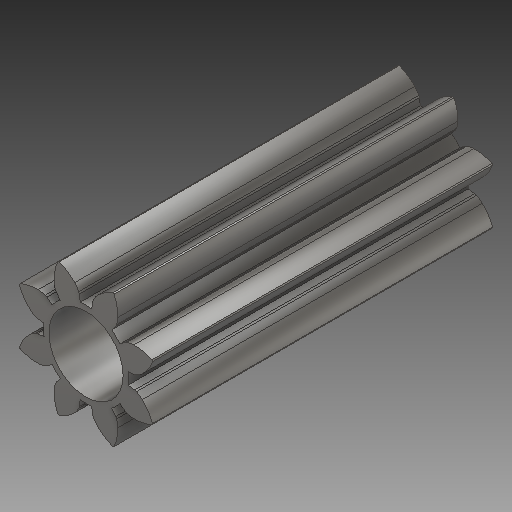
# Autodesk Inventor part: ピニオン8
Saved by Autodesk Inventor 2020 (Build 240168000, 168)
## iProperties
Created: 2018-09-09
Part Number: ピニオン8
Material: 鋼、炭素鋼
Document SubType Name: Modeling
Designer: 雪村
Density: 7.85 g/cm^3
Appearance: 半つや出し
Mass: 0.86128 g
Surface Area: 4.58108 cm^2
Volume: 0.109717 cm^3
Author: 雪村
Autodesk Inventor part; units mm, degrees
ref_plane "YZ Plane" through (0, 0, 0) normal (1, 0, 0) x (0, 1, 0)
ref_plane "XZ Plane" through (0, 0, 0) normal (0, 1, 0) x (-1, 0, 0)
ref_plane "XY Plane" through (0, 0, 0) normal (0, 0, 1) x (1, 0, 0)
sketch "スケッチ1" plane through (0, 0, 0) normal (0, 0, 1) x (1, 0, 0)
  arc A0 (-4.3849, 83.0601) -> (-4.408, 82.9909) centre (-4.1206, 82.9335) ccw
  arc A1 (-4.2334, 83.2827) -> (-4.3849, 83.0601) centre (-3.6288, 82.7082) ccw
  arc A2 (-3.6386, 83.6726) -> (-4.2334, 83.2827) centre (-3.1026, 82.2065) ccw
  arc A3 (-5.8318, 82.6909) -> (-5.7992, 82.6257) centre (-5.5555, 82.7883) ccw
  arc A4 (-5.8821, 82.9554) -> (-5.8318, 82.6909) centre (-5.0484, 82.9767) ccw
  arc A5 (-5.7372, 83.6517) -> (-5.8821, 82.9554) centre (-4.3215, 82.994) ccw
  arc A6 (-6.5939, 81.4067) -> (-6.5247, 81.3836) centre (-6.4673, 81.6709) ccw
  arc A7 (-6.8165, 81.5582) -> (-6.5939, 81.4067) centre (-6.242, 82.1627) ccw
  arc A8 (-7.2064, 82.153) -> (-6.8165, 81.5582) centre (-5.7403, 82.6889) ccw
  arc A9 (-6.2247, 79.9597) -> (-6.1595, 79.9923) centre (-6.3221, 80.2361) ccw
  arc A10 (-6.4892, 79.9095) -> (-6.2247, 79.9597) centre (-6.5105, 80.7432) ccw
  arc A11 (-7.1855, 80.0543) -> (-6.4892, 79.9095) centre (-6.5278, 81.4701) ccw
  arc A12 (-4.9405, 79.1977) -> (-4.9174, 79.2668) centre (-5.2047, 79.3242) ccw
  arc A13 (-5.092, 78.9751) -> (-4.9405, 79.1977) centre (-5.6965, 79.5495) ccw
  arc A14 (-5.6868, 78.5852) -> (-5.092, 78.9751) centre (-6.2228, 80.0513) ccw
  arc A15 (-3.4935, 79.5669) -> (-3.5261, 79.6321) centre (-3.7699, 79.4695) ccw
  arc A16 (-3.4433, 79.3023) -> (-3.4935, 79.5669) centre (-4.277, 79.2811) ccw
  arc A17 (-3.5881, 78.6061) -> (-3.4433, 79.3023) centre (-5.0039, 79.2638) ccw
  arc A18 (-2.7315, 80.8511) -> (-2.8006, 80.8742) centre (-2.858, 80.5868) ccw
  arc A19 (-2.5089, 80.6996) -> (-2.7315, 80.8511) centre (-3.0833, 80.095) ccw
  arc A20 (-2.119, 80.1048) -> (-2.5089, 80.6996) centre (-3.5851, 79.5688) ccw
  arc A21 (-3.1007, 82.298) -> (-3.1659, 82.2654) centre (-3.0033, 82.0217) ccw
  arc A22 (-2.8361, 82.3483) -> (-3.1007, 82.298) centre (-2.8149, 81.5146) ccw
  arc A23 (-2.1399, 82.2034) -> (-2.8361, 82.3483) centre (-2.7976, 80.7877) ccw
  arc A24 (-4.9174, 82.9909) -> (-4.9405, 83.0601) centre (-5.2047, 82.9335) ccw
  arc A25 (-4.9405, 83.0601) -> (-5.092, 83.2827) centre (-5.6965, 82.7082) ccw
  arc A26 (-5.092, 83.2827) -> (-5.6868, 83.6726) centre (-6.2228, 82.2065) ccw
  arc A27 (-6.1595, 82.2654) -> (-6.2247, 82.298) centre (-6.3221, 82.0217) ccw
  arc A28 (-6.2247, 82.298) -> (-6.4892, 82.3483) centre (-6.5105, 81.5146) ccw
  arc A29 (-6.4892, 82.3483) -> (-7.1855, 82.2034) centre (-6.5278, 80.7877) ccw
  arc A30 (-6.5247, 80.8742) -> (-6.5939, 80.8511) centre (-6.4673, 80.5868) ccw
  arc A31 (-6.5939, 80.8511) -> (-6.8165, 80.6996) centre (-6.242, 80.095) ccw
  arc A32 (-6.8165, 80.6996) -> (-7.2064, 80.1048) centre (-5.7403, 79.5688) ccw
  arc A33 (-5.7992, 79.6321) -> (-5.8318, 79.5669) centre (-5.5555, 79.4695) ccw
  arc A34 (-5.8318, 79.5669) -> (-5.8821, 79.3023) centre (-5.0484, 79.2811) ccw
  arc A35 (-5.8821, 79.3023) -> (-5.7372, 78.6061) centre (-4.3215, 79.2638) ccw
  arc A36 (-4.408, 79.2668) -> (-4.3849, 79.1977) centre (-4.1206, 79.3242) ccw
  arc A37 (-4.3849, 79.1977) -> (-4.2334, 78.9751) centre (-3.6288, 79.5495) ccw
  arc A38 (-4.2334, 78.9751) -> (-3.6386, 78.5852) centre (-3.1026, 80.0513) ccw
  arc A39 (-3.1659, 79.9923) -> (-3.1007, 79.9597) centre (-3.0033, 80.2361) ccw
  arc A40 (-3.1007, 79.9597) -> (-2.8361, 79.9095) centre (-2.8149, 80.7432) ccw
  arc A41 (-2.8361, 79.9095) -> (-2.1399, 80.0543) centre (-2.7976, 81.4701) ccw
  arc A42 (-2.8006, 81.3836) -> (-2.7315, 81.4067) centre (-2.858, 81.6709) ccw
  arc A43 (-2.7315, 81.4067) -> (-2.5089, 81.5582) centre (-3.0833, 82.1627) ccw
  arc A44 (-2.5089, 81.5582) -> (-2.119, 82.153) centre (-3.5851, 82.6889) ccw
  arc A45 (-3.5261, 82.6257) -> (-3.4935, 82.6909) centre (-3.7699, 82.7883) ccw
  arc A46 (-3.4935, 82.6909) -> (-3.4433, 82.9554) centre (-4.277, 82.9767) ccw
  arc A47 (-3.4433, 82.9554) -> (-3.5881, 83.6517) centre (-5.0039, 82.994) ccw
  arc A48 (-4.4424, 82.7389) -> (-4.8829, 82.7389) centre (-4.6627, 81.1289) ccw
  arc A49 (-5.6454, 82.4231) -> (-5.9569, 82.1116) centre (-4.6627, 81.1289) ccw
  arc A50 (-6.2727, 81.3491) -> (-6.2727, 80.9086) centre (-4.6627, 81.1289) ccw
  arc A51 (-5.9569, 80.1462) -> (-5.6454, 79.8347) centre (-4.6627, 81.1289) ccw
  arc A52 (-4.8829, 79.5189) -> (-4.4424, 79.5189) centre (-4.6627, 81.1289) ccw
  arc A53 (-3.68, 79.8347) -> (-3.3685, 80.1462) centre (-4.6627, 81.1289) ccw
  arc A54 (-3.0527, 80.9086) -> (-3.0527, 81.3491) centre (-4.6627, 81.1289) ccw
  arc A55 (-3.3685, 82.1116) -> (-3.68, 82.4231) centre (-4.6627, 81.1289) ccw
  arc A56 (-5.6868, 83.6726) -> (-5.7372, 83.6517) centre (-4.6627, 81.1289) ccw
  arc A57 (-7.1855, 82.2034) -> (-7.2064, 82.153) centre (-4.6627, 81.1289) ccw
  arc A58 (-7.2064, 80.1048) -> (-7.1855, 80.0543) centre (-4.6627, 81.1289) ccw
  arc A59 (-5.7372, 78.6061) -> (-5.6868, 78.5852) centre (-4.6627, 81.1289) ccw
  arc A60 (-3.6386, 78.5852) -> (-3.5881, 78.6061) centre (-4.6627, 81.1289) ccw
  arc A61 (-2.1399, 80.0543) -> (-2.119, 80.1048) centre (-4.6627, 81.1289) ccw
  arc A62 (-2.119, 82.153) -> (-2.1399, 82.2034) centre (-4.6627, 81.1289) ccw
  arc A63 (-3.5881, 83.6517) -> (-3.6386, 83.6726) centre (-4.6627, 81.1289) ccw
  line L0 (-4.4424, 82.7389) -> (-4.408, 82.9909)
  line L1 (-5.6454, 82.4231) -> (-5.7992, 82.6257)
  line L2 (-6.2727, 81.3491) -> (-6.5247, 81.3836)
  line L3 (-5.9569, 80.1462) -> (-6.1595, 79.9923)
  line L4 (-4.8829, 79.5189) -> (-4.9174, 79.2668)
  line L5 (-3.68, 79.8347) -> (-3.5261, 79.6321)
  line L6 (-3.0527, 80.9086) -> (-2.8006, 80.8742)
  line L7 (-3.3685, 82.1116) -> (-3.1659, 82.2654)
  line L8 (-4.8829, 82.7389) -> (-4.9174, 82.9909)
  line L9 (-5.9569, 82.1116) -> (-6.1595, 82.2654)
  line L10 (-6.2727, 80.9086) -> (-6.5247, 80.8742)
  line L11 (-5.6454, 79.8347) -> (-5.7992, 79.6321)
  line L12 (-4.4424, 79.5189) -> (-4.408, 79.2668)
  line L13 (-3.3685, 80.1462) -> (-3.1659, 79.9923)
  line L14 (-3.0527, 81.3491) -> (-2.8006, 81.3836)
  line L15 (-3.68, 82.4231) -> (-3.5261, 82.6257)
  line L16 (-9.4048, 81.1289) -> (0.0794, 81.1289)
  line L17 (-4.6627, 76.3867) -> (-4.6627, 85.871)
  line L18 (18.0795, 83.871) -> (88.0795, 83.871)
  line L19 (18.0795, 75.871) -> (88.0795, 75.871)
  line L20 (18.0795, 67.871) -> (88.0795, 67.871)
  line L21 (18.0795, 59.871) -> (88.0795, 59.871)
  line L22 (18.0795, 51.871) -> (88.0795, 51.871)
  line L23 (18.0795, 43.871) -> (88.0795, 43.871)
  line L24 (18.0795, 35.871) -> (88.0795, 35.871)
  line L25 (18.0795, 27.871) -> (88.0795, 27.871)
  line L26 (18.0795, 19.871) -> (88.0795, 19.871)
  line L27 (18.0795, 11.871) -> (88.0795, 11.871)
  line L28 (18.0795, 3.871) -> (88.0795, 3.871)
  line L29 (18.0795, -4.129) -> (88.0795, -4.129)
  line L30 (18.0795, -12.129) -> (88.0795, -12.129)
  line L31 (18.0795, 83.871) -> (18.0795, -12.129)
  line L32 (88.0795, 83.871) -> (88.0795, -12.129)
  line L33 (53.0795, 75.871) -> (53.0795, -12.129)
  point P0 (0, 0)
  point P1 (24.0795, 77.871)
  point P2 (26.5795, 69.871)
  point P3 (26.5795, 61.871)
  point P4 (24.0795, 53.871)
  point P5 (26.5795, 45.871)
  point P6 (21.5795, 37.871)
  point P7 (24.0795, 29.871)
  point P8 (24.0795, 21.871)
  point P9 (24.0795, 13.871)
  point P10 (26.5795, 5.871)
  point P11 (26.5795, -2.129)
  point P12 (24.0795, -10.129)
  point P13 (54.0795, 69.871)
  point P14 (70.3295, 61.871)
  point P15 (67.8295, 53.871)
  point P16 (66.5795, 45.871)
  point P17 (70.3295, 37.871)
  point P18 (64.0795, 29.871)
  point P19 (64.0795, 21.871)
  point P20 (66.5795, 13.871)
  point P21 (64.0795, 5.871)
  point P22 (-3.6627, 99.371)
  point P23 (-3.6627, 93.371)
  point P24 (14.6498, 99.371)
  point P25 (15.7123, 93.371)
  constraints: 128 point on circle, 64 centre point, 64 end point, 2 midpoint, 53 other
extrude "押し出し1" add sketch "スケッチ1" along normal blind 13 contours A1 A2 A63 A47 A46 A45 L15 A55 L7 A21 A22 A23 A62 A44 A43 A42 L14 A54 L16 L17 A48 L0 A0 | L17 L16 A50 L2 A6 A7 A8 A57 A29 A28 A27 L9 A49 L1 A3 A4 A5 A56 A26 A25 A24 L8 A48 | L17 A52 L4 A12 A13 A14 A59 A35 A34 A33 L11 A51 L3 A9 A10 A11 A58 A32 A31 A30 L10 A50 L16 | L16 A54 L6 A18 A19 A20 A61 A41 A40 A39 L13 A53 L5 A15 A16 A17 A60 A38 A37 A36 L12 A52 L17
sketch "スケッチ2" plane through (0, 0, 13) normal (0, 0, 1) x (1, 0, 0)
  arc A0 (-4.3849, 83.0601) -> (-4.408, 82.9909) centre (-4.1206, 82.9335) ccw construction
  line L0 (-4.408, 82.9909) -> (-4.4424, 82.7389) construction
  arc A1 (-4.4424, 82.7389) -> (-4.8829, 82.7389) centre (-4.6627, 81.1289) ccw construction
  line L1 (-4.8829, 82.7389) -> (-4.9174, 82.9909) construction
  arc A2 (-4.9174, 82.9909) -> (-4.9405, 83.0601) centre (-5.2047, 82.9335) ccw construction
  arc A3 (-4.9405, 83.0601) -> (-5.092, 83.2827) centre (-5.6965, 82.7082) ccw construction
  arc A4 (-5.092, 83.2827) -> (-5.6868, 83.6726) centre (-6.2228, 82.2065) ccw construction
  arc A5 (-5.6868, 83.6726) -> (-5.7372, 83.6517) centre (-4.6627, 81.1289) ccw construction
  arc A6 (-5.7372, 83.6517) -> (-5.8821, 82.9554) centre (-4.3215, 82.994) ccw construction
  arc A7 (-5.8821, 82.9554) -> (-5.8318, 82.6909) centre (-5.0484, 82.9767) ccw construction
  arc A8 (-5.8318, 82.6909) -> (-5.7992, 82.6257) centre (-5.5555, 82.7883) ccw construction
  line L2 (-5.7992, 82.6257) -> (-5.6454, 82.4231) construction
  arc A9 (-5.6454, 82.4231) -> (-5.9569, 82.1116) centre (-4.6627, 81.1289) ccw construction
  line L3 (-5.9569, 82.1116) -> (-6.1595, 82.2654) construction
  arc A10 (-6.1595, 82.2654) -> (-6.2247, 82.298) centre (-6.3221, 82.0217) ccw construction
  arc A11 (-6.2247, 82.298) -> (-6.4892, 82.3483) centre (-6.5105, 81.5146) ccw construction
  arc A12 (-6.4892, 82.3483) -> (-7.1855, 82.2034) centre (-6.5278, 80.7877) ccw construction
  arc A13 (-7.1855, 82.2034) -> (-7.2064, 82.153) centre (-4.6627, 81.1289) ccw construction
  arc A14 (-7.2064, 82.153) -> (-6.8165, 81.5582) centre (-5.7403, 82.6889) ccw construction
  arc A15 (-6.8165, 81.5582) -> (-6.5939, 81.4067) centre (-6.242, 82.1627) ccw construction
  arc A16 (-6.5939, 81.4067) -> (-6.5247, 81.3836) centre (-6.4673, 81.6709) ccw construction
  line L4 (-6.5247, 81.3836) -> (-6.2727, 81.3491) construction
  arc A17 (-6.2727, 81.3491) -> (-6.2727, 80.9086) centre (-4.6627, 81.1289) ccw construction
  line L5 (-6.2727, 80.9086) -> (-6.5247, 80.8742) construction
  arc A18 (-6.5247, 80.8742) -> (-6.5939, 80.8511) centre (-6.4673, 80.5868) ccw construction
  arc A19 (-6.5939, 80.8511) -> (-6.8165, 80.6996) centre (-6.242, 80.095) ccw construction
  arc A20 (-6.8165, 80.6996) -> (-7.2064, 80.1048) centre (-5.7403, 79.5688) ccw construction
  arc A21 (-7.2064, 80.1048) -> (-7.1855, 80.0543) centre (-4.6627, 81.1289) ccw construction
  arc A22 (-7.1855, 80.0543) -> (-6.4892, 79.9095) centre (-6.5278, 81.4701) ccw construction
  arc A23 (-6.4892, 79.9095) -> (-6.2247, 79.9597) centre (-6.5105, 80.7432) ccw construction
  arc A24 (-6.2247, 79.9597) -> (-6.1595, 79.9923) centre (-6.3221, 80.2361) ccw construction
  line L6 (-6.1595, 79.9923) -> (-5.9569, 80.1462) construction
  arc A25 (-5.9569, 80.1462) -> (-5.6454, 79.8347) centre (-4.6627, 81.1289) ccw construction
  line L7 (-5.6454, 79.8347) -> (-5.7992, 79.6321) construction
  arc A26 (-5.7992, 79.6321) -> (-5.8318, 79.5669) centre (-5.5555, 79.4695) ccw construction
  arc A27 (-5.8318, 79.5669) -> (-5.8821, 79.3023) centre (-5.0484, 79.2811) ccw construction
  arc A28 (-5.8821, 79.3023) -> (-5.7372, 78.6061) centre (-4.3215, 79.2638) ccw construction
  arc A29 (-5.7372, 78.6061) -> (-5.6868, 78.5852) centre (-4.6627, 81.1289) ccw construction
  arc A30 (-5.6868, 78.5852) -> (-5.092, 78.9751) centre (-6.2228, 80.0513) ccw construction
  arc A31 (-5.092, 78.9751) -> (-4.9405, 79.1977) centre (-5.6965, 79.5495) ccw construction
  arc A32 (-4.9405, 79.1977) -> (-4.9174, 79.2668) centre (-5.2047, 79.3242) ccw construction
  line L8 (-4.9174, 79.2668) -> (-4.8829, 79.5189) construction
  arc A33 (-4.8829, 79.5189) -> (-4.4424, 79.5189) centre (-4.6627, 81.1289) ccw construction
  line L9 (-4.4424, 79.5189) -> (-4.408, 79.2668) construction
  arc A34 (-4.408, 79.2668) -> (-4.3849, 79.1977) centre (-4.1206, 79.3242) ccw construction
  arc A35 (-4.3849, 79.1977) -> (-4.2334, 78.9751) centre (-3.6288, 79.5495) ccw construction
  arc A36 (-4.2334, 78.9751) -> (-3.6386, 78.5852) centre (-3.1026, 80.0513) ccw construction
  arc A37 (-3.6386, 78.5852) -> (-3.5881, 78.6061) centre (-4.6627, 81.1289) ccw construction
  arc A38 (-3.5881, 78.6061) -> (-3.4433, 79.3023) centre (-5.0039, 79.2638) ccw construction
  arc A39 (-3.4433, 79.3023) -> (-3.4935, 79.5669) centre (-4.277, 79.2811) ccw construction
  arc A40 (-3.4935, 79.5669) -> (-3.5261, 79.6321) centre (-3.7699, 79.4695) ccw construction
  line L10 (-3.5261, 79.6321) -> (-3.68, 79.8347) construction
  arc A41 (-3.68, 79.8347) -> (-3.3685, 80.1462) centre (-4.6627, 81.1289) ccw construction
  line L11 (-3.3685, 80.1462) -> (-3.1659, 79.9923) construction
  arc A42 (-3.1659, 79.9923) -> (-3.1007, 79.9597) centre (-3.0033, 80.2361) ccw construction
  arc A43 (-3.1007, 79.9597) -> (-2.8361, 79.9095) centre (-2.8149, 80.7432) ccw construction
  arc A44 (-2.8361, 79.9095) -> (-2.1399, 80.0543) centre (-2.7976, 81.4701) ccw construction
  arc A45 (-2.1399, 80.0543) -> (-2.119, 80.1048) centre (-4.6627, 81.1289) ccw construction
  arc A46 (-2.119, 80.1048) -> (-2.5089, 80.6996) centre (-3.5851, 79.5688) ccw construction
  arc A47 (-2.5089, 80.6996) -> (-2.7315, 80.8511) centre (-3.0833, 80.095) ccw construction
  arc A48 (-2.7315, 80.8511) -> (-2.8006, 80.8742) centre (-2.858, 80.5868) ccw construction
  line L12 (-2.8006, 80.8742) -> (-3.0527, 80.9086) construction
  arc A49 (-3.0527, 80.9086) -> (-3.0527, 81.3491) centre (-4.6627, 81.1289) ccw construction
  line L13 (-3.0527, 81.3491) -> (-2.8006, 81.3836) construction
  arc A50 (-2.8006, 81.3836) -> (-2.7315, 81.4067) centre (-2.858, 81.6709) ccw construction
  arc A51 (-2.7315, 81.4067) -> (-2.5089, 81.5582) centre (-3.0833, 82.1627) ccw construction
  arc A52 (-2.5089, 81.5582) -> (-2.119, 82.153) centre (-3.5851, 82.6889) ccw construction
  arc A53 (-2.119, 82.153) -> (-2.1399, 82.2034) centre (-4.6627, 81.1289) ccw construction
  arc A54 (-2.1399, 82.2034) -> (-2.8361, 82.3483) centre (-2.7976, 80.7877) ccw construction
  arc A55 (-2.8361, 82.3483) -> (-3.1007, 82.298) centre (-2.8149, 81.5146) ccw construction
  arc A56 (-3.1007, 82.298) -> (-3.1659, 82.2654) centre (-3.0033, 82.0217) ccw construction
  line L14 (-3.1659, 82.2654) -> (-3.3685, 82.1116) construction
  arc A57 (-3.3685, 82.1116) -> (-3.68, 82.4231) centre (-4.6627, 81.1289) ccw construction
  line L15 (-3.68, 82.4231) -> (-3.5261, 82.6257) construction
  arc A58 (-3.5261, 82.6257) -> (-3.4935, 82.6909) centre (-3.7699, 82.7883) ccw construction
  arc A59 (-3.4935, 82.6909) -> (-3.4433, 82.9554) centre (-4.277, 82.9767) ccw construction
  arc A60 (-3.4433, 82.9554) -> (-3.5881, 83.6517) centre (-5.0039, 82.994) ccw construction
  arc A61 (-3.5881, 83.6517) -> (-3.6386, 83.6726) centre (-4.6627, 81.1289) ccw construction
  arc A62 (-3.6386, 83.6726) -> (-4.2334, 83.2827) centre (-3.1026, 82.2065) ccw construction
  arc A63 (-4.2334, 83.2827) -> (-4.3849, 83.0601) centre (-3.6288, 82.7082) ccw construction
  circle A64 centre (-4.6627, 81.1289) radius 1.42
  point P0 (0, 0)
  dimension "d2" = 2.84
  constraints: 1 centre point, 1 coincident
  measures "d2" diameter of A64
extrude "押し出し2" cut sketch "スケッチ2" against normal through all
